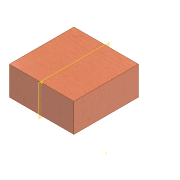
# Autodesk Inventor part: abb
Saved by Autodesk Inventor 2021 (Build 250183000, 183)
## iProperties
Created: 2021-07-07
Part Number: abb
Material: Generic
Document SubType Name: Modeling
Designer: Shaheen Khan
Density: 1 g/cm^3
Appearance: Walnut - Natural Polished
Author: Shaheen Khan
Autodesk Inventor part; units mm, degrees
ref_plane "XZ Plane" through (0, 0, 0) normal (0, 1, 0) x (-1, 0, 0)
ref_plane "XY Plane" through (0, 0, 0) normal (0, 0, 1) x (1, 0, 0)
sketch "Sketch1" plane through (0, 0, 0) normal (0, 1, 0) x (-1, 0, 0)
  line L0 (0, 0) -> (90, 0)
  line L1 (90, 0) -> (90, -90)
  line L2 (90, -90) -> (0, -90)
  line L3 (0, -90) -> (0, 0)
  dimension "d0" = 90
  dimension "d1" = 90
  constraints: 8 end point, 2 parallel, 1 horizontal, 1 perpendicular
  measures "d0" distance of L2.end L0.start
  measures "d1" distance of L0.start L0.end
extrude "Extrusion1" add sketch "Sketch1" along normal blind 40
ref_plane "Work Plane1" through (45, 0, 0) normal (1, 0, 0) x (0, 0, -1)
ref_plane "Work Plane2" through (-45, 0, 0) normal (1, 0, 0) x (0, 1, 0)
sketch "Sketch2" plane through (45, 0, 0) normal (1, 0, 0) x (0, 0, -1)
  point P0 (0, 0)
body "Solid1"
